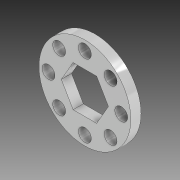
# Autodesk Inventor part: Gobilda Mechanum .5 in Hex Hub (drilled out wheel)
Saved by Autodesk Inventor 2022 (Build 260153000, 153)
## iProperties
Created: 2021-08-29
Part Number: Gobilda Mechanum .5 in Hex Hub (drilled out wheel)
Material: Aluminum 6061
Document SubType Name: Modeling
Density: 2.7 g/cm^3
Appearance: Aluminum - Dark
Autodesk Inventor part; units mm, degrees
ref_plane "YZ Plane" through (0, 0, 0) normal (1, 0, 0) x (0, 1, 0)
ref_plane "XZ Plane" through (0, 0, 0) normal (0, 1, 0) x (-1, 0, 0)
ref_plane "XY Plane" through (0, 0, 0) normal (0, 0, 1) x (1, 0, 0)
sketch "Sketch1" plane through (0, 0, 0) normal (0, 0, 1) x (1, 0, 0)
  line L0 (3.6662, 6.35) -> (7.3323, 0)
  line L1 (7.3323, 0) -> (3.6662, -6.35)
  line L2 (3.6662, -6.35) -> (-3.6662, -6.35)
  line L3 (-3.6662, -6.35) -> (-7.3323, 0)
  line L4 (-7.3323, 0) -> (-3.6662, 6.35)
  line L5 (-3.6662, 6.35) -> (3.6662, 6.35)
  circle A0 centre (0, 11.3137) radius 2
  circle A1 centre (-8, 8) radius 2
  circle A2 centre (-11.3137, 0) radius 2
  circle A3 centre (-8, -8) radius 2
  circle A4 centre (0, -11.3137) radius 2
  circle A5 centre (8, -8) radius 2
  circle A6 centre (11.3137, 0) radius 2
  circle A7 centre (8, 8) radius 2
  circle A8 centre (0, 0) radius 14.2875
  dimension "d0" = 12.7
  dimension "d1" = 4
  dimension "d4" = 360
  dimension "d6" = 16
  dimension "d7" = 28.575
  constraints: 12 end point, 9 centre point, 2 coincident, 1 horizontal, 1 vertical alignment, 30 other
  measures "d0" distance between parallel lines of L2 L5
  measures "d1" diameter of A0
  measures "d6" distance of A6.centre A0.centre
  measures "d7" diameter of A8
extrude "Extrusion1" add sketch "Sketch1" along normal blind 3.175
body "Solid1"
